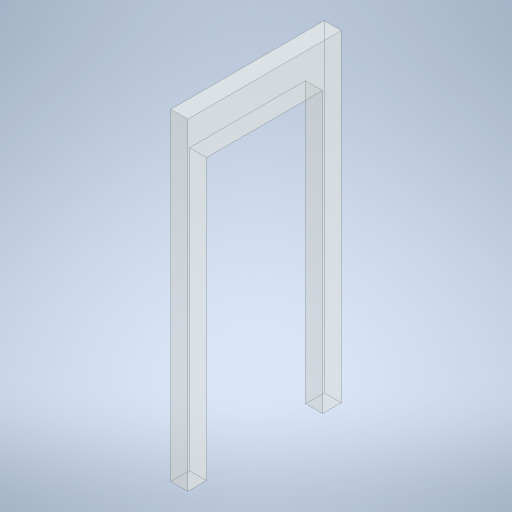
# Autodesk Inventor part: Wall_With_Door_For_Attic_Room
Saved by Autodesk Inventor 2024 (Build 280153000, 153)
## iProperties
Created: 2023-05-20
Part Number: Wall_With_Door_For_Attic_Room
Material: Wood (Southern Pine)
Document SubType Name: Modeling
Designer: Tom
Density: 0.420735 g/cm^3
Appearance: Clear
Author: Tom
Autodesk Inventor part; units mm, degrees
ref_plane "YZ Plane" through (0, 0, 0) normal (1, 0, 0) x (0, 1, 0)
ref_plane "XZ Plane" through (0, 0, 0) normal (0, 1, 0) x (-1, 0, 0)
ref_plane "XY Plane" through (0, 0, 0) normal (0, 0, 1) x (1, 0, 0)
sketch "Sketch1" plane through (0, 0, 0) normal (1, 0, 0) x (0, 1, 0)
  line L0 (0, 0) -> (2400.3, 0)
  line L1 (2400.3, 0) -> (2400.3, -1143)
  line L2 (2400.3, -1143) -> (0, -1143)
  line L3 (0, -1143) -> (0, 0)
  dimension "d0" = 1143
  dimension "d1" = 2400.3
  constraints: 8 end point, 2 parallel, 1 horizontal, 1 perpendicular
  measures "d0" distance of L2.end L0.start
  measures "d1" distance of L0.start L0.end
extrude "Extrusion1" add sketch "Sketch1" along normal blind 127
sketch "Sketch2" plane through (127, 0, 0) normal (1, 0, 0) x (0, 0, -1)
  line L0 (0, 0) -> (1143, 0) projected
  line L1 (1003.3, 0) -> (139.7, 0)
  line L2 (139.7, 0) -> (139.7, 2082.8)
  line L3 (139.7, 2082.8) -> (1003.3, 2082.8)
  line L4 (1003.3, 2082.8) -> (1003.3, 0)
  line L5 (1143, 0) -> (1143, 2400.3) projected
  dimension "d4" = 2082.8
  dimension "d6" = 139.7
  dimension "d7" = 863.6
  constraints: 8 end point, 2 parallel, 1 horizontal, 1 perpendicular, 1 point on line
  measures "d4" distance of L1.end L2.end
  measures "d6" distance between parallel lines of L5 L4
  measures "d7" distance of L1.start L1.end
extrude "Extrusion2" cut sketch "Sketch2" against normal up to surface (127 mm away)
body "Solid1"
